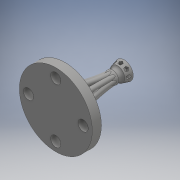
# Autodesk Inventor part: Design 2
Saved by Autodesk Inventor 2017 (Build 210142000, 142)
## iProperties
Created: 2019-10-23
Part Number: Design 2
Material: 3D Printed Steel
Document SubType Name: Modeling
Designer: aquin
Density: 8 g/cm^3
Appearance: Generic
Mass: 30.966 g
Surface Area: 33.9153 cm^2
Volume: 3.87075 cm^3
Author: aquin
Autodesk Inventor part; units mm, degrees
sketch "Sketch1" plane through (0, 0, 0) normal (0, 0, 1) x (1, 0, 0)
  line L0 (0, 0) -> (16, 0)
  line L1 (16, 0) -> (16, 4)
  line L2 (16, 0) -> (20, 0) construction
  line L3 (16, 4) -> (8, 4)
  line L4 (0, 0) -> (0, 30)
  line L5 (0, 30) -> (4, 30)
  line L6 (4, 30) -> (8, 4)
  dimension "d0" = 16
  dimension "d1" = 4
  dimension "d2" = 90
  dimension "d3" = 8
  dimension "d4" = 30
  dimension "d5" = 4
  constraints: 14 end point, 3 perpendicular, 2 horizontal, 2 vertical
  measures "d0" distance of L0.start L0.end
  measures "d1" distance of L0.end L1.end
  measures "d2" angle of L2 L1
  measures "d3" distance of L1.end L3.end
  measures "d4" distance of L0.start L4.end
  measures "d5" distance of L4.end L5.end
revolve "Revolution1" add sketch "Sketch1" angle 360 about axis through (0, 0, 0) along (0, 1, 0)
sketch "Sketch2" plane through (0, 4, 0) normal (0, 1, 0) x (1, 0, 0)
  circle A0 centre (0, 0) radius 16 projected
  line L0 (0, 0) -> (0, 12)
  line L1 (0, 12) -> (-12, 12)
  line L2 (-12, 12) -> (-12, 0)
  circle A1 centre (0, 0) radius 4 projected
  line L3 (0, 0) -> (12, 0)
  line L4 (12, 0) -> (12, -12)
  line L5 (12, -12) -> (0, -12)
  dimension "d7" = 12
  dimension "d8" = 12
  dimension "d9" = 90
  dimension "d10" = 12
  dimension "d11" = 12
  dimension "d12" = 12
  dimension "d13" = 90
  constraints: 12 end point, 4 perpendicular, 1 horizontal, 1 vertical
  measures "d7" distance of L0.start L0.end
  measures "d8" distance of L0.end L1.end
  measures "d9" angle of L1 L0
  measures "d10" distance of L1.end L2.end
  measures "d11" distance of L3.start L3.end
  measures "d12" distance of L3.end L4.end
  measures "d13" angle of L3 L4
hole "Hole1" at (-12, 4, 0) at (0, 4, -12) at (12, 4, 0) at (0, 4, 12) direction (0, -1, 0) diameter 4.5 depth 8 tip angle 118
sketch "Sketch3" plane through (0, 4, 0) normal (0, 1, 0) x (1, 0, 0)
  circle A0 centre (0, 0) radius 4
  circle A1 centre (0, 0) radius 8
  constraints: 2 centre point, 2 coincident
extrude "Extrusion1" cut sketch "Sketch3" along normal blind 28.75
sketch "Sketch4" plane through (0, 0, 0) normal (1, 0, 0) x (0, 1, 0)
  line L0 (4, 4) -> (30, 4) projected
  arc A0 (4, 4) -> (30, 4) centre (17, 47.0813) ccw
  line L1 (-6, 0) -> (36, 0) projected
  point P0 (0, 0)
  dimension "d23" = 45
  constraints: 2 point on circle, 2 point on line, 1 centre point
  measures "d23" radius of A0
revolve "Revolution2" cut sketch "Sketch4" angle 360 about axis through (0, -10, 0) along (0, 1, 0)
sketch "Sketch5" plane through (0, 4, 0) normal (0, 1, 0) x (1, 0, 0)
  line L0 (0, 0) -> (0, -8)
  dimension "d25" = 8
  constraints: 2 end point, 1 vertical
  measures "d25" distance of L0.start L0.end
ref_plane "Work Plane1" through (0, 4, 0) normal (-0.1736, 0.9848, 0) x (0, 0, 1)
sketch "Sketch6" plane through (0, 4, 0) normal (0, 1, 0) x (1, 0, 0)
  line L0 (0, 0) -> (8, 0)
  dimension "d27" = 8
  constraints: 2 end point, 1 horizontal
  measures "d27" distance of L0.start L0.end
ref_plane "Work Plane2" through (0.2605, 2.5228, 0) normal (-0.1736, 0.9848, 0) x (0, 0, 1)
sketch "Sketch8" plane through (0.2605, 2.5228, 0) normal (-0.1736, 0.9848, 0) x (0, 0, 1)
  circle A0 centre (0, 6) radius 1
  point P0 (0, -0.6946)
  dimension "d39" = 2
  constraints: 1 centre point
  measures "d39" diameter of A0
sketch "Sketch9" plane through (0, 0, 0) normal (0, 0, 1) x (1, 0, 0)
  arc A0 (4, 30) -> (4, 4) centre (47.0813, 17) ccw projected
  arc A1 (1.6574, 24.4102) -> (6.1856, 3.5632) centre (69.5862, 28.25) ccw
  point P0 (0, 0)
  constraints: 2 point on circle, 1 centre point
sweep "Sweep2" add profiles "Sketch8" path "Sketch9" path curves A1
pattern_circular "Circular Pattern2" count 8 over 360 about axis through (0, -10, 0) along (0, 1, 0) of "Sweep2"
ref_plane "Work Plane4" through (0, 1.693, -4.9167) normal (0, -0.3256, 0.9455) x (1, 0, 0)
ref_plane "Work Plane3" through (0, 0, 0) normal (0, -0.3256, 0.9455) x (1, 0, 0)
sketch "Sketch10" plane through (0, 1.693, -4.9167) normal (0, -0.3256, 0.9455) x (1, 0, 0)
  line L0 (0, 4.357) -> (0.872, 3.7235)
  line L1 (0.872, 3.7235) -> (0.5389, 2.6983)
  line L2 (0.5389, 2.6983) -> (-0.5389, 2.6983)
  line L3 (-0.5389, 2.6983) -> (-0.872, 3.7235)
  line L4 (-0.872, 3.7235) -> (0, 4.357)
  point P0 (0, 0)
  point P1 (0, 3.4401)
  constraints: 10 end point, 11 other
extrude "Extrusion3" cut sketch "Sketch10" along normal blind 3
pattern_circular "Circular Pattern3" count 8 over 360 about axis through (0, -10, 0) along (0, 1, 0) of "Extrusion3"
ref_plane "Work Plane6" through (0, 0.7814, -4.4316) normal (0, -0.1736, 0.9848) x (1, 0, 0)
ref_plane "Work Plane5" through (0, 0, 0) normal (0, -0.1736, 0.9848) x (1, 0, 0)
sketch "Sketch11" plane through (0, 0.7814, -4.4316) normal (0, -0.1736, 0.9848) x (1, 0, 0)
  line L0 (0, 6.3299) -> (0, 4.8773) projected
  line L1 (0, 7.1365) -> (0.7672, 6.5791)
  line L2 (0.7672, 6.5791) -> (0.4741, 5.6772)
  line L3 (0.4741, 5.6772) -> (-0.4741, 5.6772)
  line L4 (-0.4741, 5.6772) -> (-0.7672, 6.5791)
  line L5 (-0.7672, 6.5791) -> (0, 7.1365)
  point P0 (0, 0)
  constraints: 10 end point, 11 other
extrude "Extrusion4" cut sketch "Sketch11" along normal blind 3
pattern_circular "Circular Pattern4" count 4 over 360 about axis through (0, -10, 0) along (0, 1, 0) of "Extrusion4"
ref_plane "Work Plane7" through (0, 0.2171, -1.231) normal (0, -0.1736, 0.9848) x (1, 0, 0)
sketch "Sketch12" plane through (0, 0.2171, -1.231) normal (0, -0.1736, 0.9848) x (1, 0, 0)
  ellipse E0 centre (0, 29.5442) end of major axis (4, 29.5442) minor radius 0.6946 projected
  line L0 (0, 29.5442) -> (0.8712, 28.9113)
  line L1 (0.8712, 28.9113) -> (0.5384, 27.8871)
  line L2 (0.5384, 27.8871) -> (-0.5384, 27.8871)
  line L3 (-0.5384, 27.8871) -> (-0.8712, 28.9113)
  line L4 (-0.8712, 28.9113) -> (0, 29.5442)
  point P0 (0, 0)
  point P1 (0, 28.6282)
  constraints: 10 end point, 12 other
extrude "Extrusion5" cut sketch "Sketch12" against normal blind 2 contours L3 L4 L0 L1 E0 | E0 L1 L2 L3 picked at (0.434, 29.103)
pattern_circular "Circular Pattern5" count 8 over 360 about axis through (0, -10, 0) along (0, 1, 0) of "Extrusion5"
sketch "Sketch13" plane through (0, 0, 0) normal (1, 0, 0) x (0, 1, 0)
  arc A0 (24.0922, 2.6437) -> (30, 4) centre (17, 47.0813) ccw projected
  line L0 (-6.0046, 0) -> (36.0274, 0) projected
  arc A1 (24.8287, 2.7675) -> (27.0566, 3.2194) centre (25.8357, 3.5209) ccw
  point P0 (0, 0)
  constraints: 4 point on circle, 1 centre point
revolve "Revolution3" cut sketch "Sketch13" angle 360 about axis through (0, -10, 0) along (0, 1, 0)
body "Solid1"
